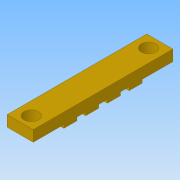
# Autodesk Inventor part: ContactPress
Saved by Autodesk Inventor 2017.3 (Build 213256000, 256)
## iProperties
Created: 2019-06-22
Part Number: ContactPress
Material: ABS Plastic
Document SubType Name: Modeling
Designer: Derek Wider
Density: 1.06 g/cm^3
Appearance: Gold
Author: Derek Wider
Autodesk Inventor part; units mm, degrees
ref_plane "YZ Plane" through (0, 0, 0) normal (1, 0, 0) x (0, 1, 0)
ref_plane "XZ Plane" through (0, 0, 0) normal (0, 1, 0) x (-1, 0, 0)
ref_plane "XY Plane" through (0, 0, 0) normal (0, 0, 1) x (1, 0, 0)
sketch "Sketch1" plane through (0, 0, 0) normal (0, 1, 0) x (-1, 0, 0)
  line L0 (0, 0) -> (6.096, 0)
  line L1 (6.096, 0) -> (6.096, -32.6136)
  line L2 (6.096, -32.6136) -> (0, -32.6136)
  line L3 (0, -32.6136) -> (0, 0)
  dimension "d0" = 6.096
  dimension "d1" = 32.6136
  constraints: 8 end point, 2 parallel, 1 horizontal, 1 perpendicular
  measures "d0" distance of L1.end L2.end
  measures "d1" distance of L0.end L1.end
extrude "Extrusion1" add sketch "Sketch1" along normal blind 2.54
sketch "Sketch2" plane through (0, 0, 0) normal (0, -1, 0) x (1, 0, 0)
  line L0 (0, 0) -> (0, -32.6136) projected
  line L1 (0, -7.1628) -> (-6.096, -7.1628)
  line L2 (-6.096, -7.1628) -> (-6.096, -10.2108)
  line L3 (-6.096, -10.2108) -> (0, -10.2108)
  line L4 (0, -10.2108) -> (0, -7.1628)
  line L5 (0, -12.2428) -> (-6.096, -12.2428)
  line L6 (-6.096, -12.2428) -> (-6.096, -15.2908)
  line L7 (-6.096, -15.2908) -> (0, -15.2908)
  line L8 (0, -15.2908) -> (0, -12.2428)
  line L9 (0, -17.3228) -> (-6.096, -17.3228)
  line L10 (-6.096, -17.3228) -> (-6.096, -20.3708)
  line L11 (-6.096, -20.3708) -> (0, -20.3708)
  line L12 (0, -20.3708) -> (0, -17.3228)
  line L13 (0, -22.4028) -> (-6.096, -22.4028)
  line L14 (-6.096, -22.4028) -> (-6.096, -25.4508)
  line L15 (-6.096, -25.4508) -> (0, -25.4508)
  line L16 (0, -25.4508) -> (0, -22.4028)
  line L17 (-3.048, -10.2108) -> (-3.048, -12.2428) construction
  line L18 (-3.048, -15.2908) -> (-3.048, -17.3228) construction
  line L19 (-3.048, -20.3708) -> (-3.048, -22.4028) construction
  line L20 (-6.096, 0) -> (-6.096, -32.6136) construction
  line L21 (-6.096, 0) -> (0, 0) construction
  line L22 (0, -7.1628) -> (0, 0) construction
  line L23 (0, -32.6136) -> (0, -25.4508) construction
  dimension "d4" = 3.048
  dimension "d13" = 2.032
  constraints: 42 end point, 8 parallel, 7 collinear, 6 midpoint, 6 point on line, 5 perpendicular, 4 horizontal, 3 vertical alignment
  measures "d4" distance between parallel lines of L1 L3
  measures "d13" distance of L17.start L17.end
extrude "Extrusion2" add sketch "Sketch2" along normal blind 0.762
sketch "Sketch3" plane through (0, 0, 0) normal (0, -1, 0) x (1, 0, 0)
  line L0 (0, -7.1628) -> (-6.096, -7.1628) construction
  line L1 (-6.096, -7.1628) -> (-6.096, -10.2108) construction
  line L2 (-6.096, -10.2108) -> (0, -10.2108) construction
  line L3 (0, -10.2108) -> (0, -7.1628) construction
  line L4 (0, -22.4028) -> (-6.096, -22.4028) construction
  line L5 (-6.096, -22.4028) -> (-6.096, -25.4508) construction
  line L6 (-6.096, -25.4508) -> (0, -25.4508) construction
  line L7 (0, -25.4508) -> (0, -22.4028) construction
  circle A0 centre (-3.048, -2.5908) radius 1.7145
  circle A1 centre (-3.048, -30.0228) radius 1.7145
  line L8 (0, -7.1628) -> (-6.096, -7.1628) projected
  line L9 (-6.096, -25.4508) -> (0, -25.4508) projected
  point P0 (0, 0)
  point P1 (-3.048, -7.1628)
  point P2 (-3.048, -25.4508)
  dimension "d7" = 4.572
  dimension "d8" = 4.572
  dimension "d9" = 3.429
  dimension "d10" = 3.429
  constraints: 2 centre point, 2 midpoint, 2 vertical alignment
  measures "d7" distance from line of L0 A0.centre
  measures "d8" distance from line of L6 A1.centre
  measures "d9" diameter of A0
  measures "d10" diameter of A1
extrude "Extrusion3" cut sketch "Sketch3" against normal through all
equation "\"d8\" = d7"
equation "\"d10\" = d9"
body "Solid1"
